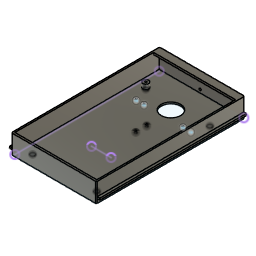
new_Backplate v28 (Autodesk Fusion 360 design; units mm, degrees)
Autodesk Fusion 360 part; units mm, degrees
sketch "Sketch1" plane through (0, 0, 0) normal (0, 0, 1) x (1, 0, 0)
  line L0 (0, 0) -> (109, 0)
  line L1 (109, 0) -> (109, 190)
  line L2 (109, 190) -> (0, 190)
  line L3 (0, 190) -> (0, 0)
  dimension "d1" = 190
  dimension "d2" = 109
  constraint horizontal L0
  constraint vertical L1
  constraint horizontal L2
  constraint vertical L3
  constraint coincident L0.start L3.end
  measures "d1" distance of L0.start L2.end
  measures "d2" distance of L0.start L0.end
extrude "Extrude1" add sketch "Sketch1" along normal blind 18.5 makes body 1
sketch "Sketch2" plane through (0, 0, 18.5) normal (0, 0, 1) x (-1, 0, 0)
  line L0 (0, -190) -> (0, 0)
  line L1 (0, 0) -> (-109, 0)
  line L2 (-109, 0) -> (-109, -190)
  line L3 (-109, -190) -> (0, -190)
  line L4 (-2, -187.5) -> (-107, -187.5)
  line L5 (-107, -187.5) -> (-107, -2.5)
  line L6 (-107, -2.5) -> (-2, -2.5)
  line L7 (-2, -2.5) -> (-2, -187.5)
  dimension "d5" = 2.5
  dimension "d6" = 2.5
  dimension "d7" = 2
  dimension "d8" = 2
  constraint horizontal L4
  constraint vertical L5
  constraint horizontal L6
  constraint vertical L7
  measures "d5" distance of L3 L4
  measures "d6" distance of L1 L6
  measures "d7" distance of L0 L7
  measures "d8" distance of L2 L5
extrude "Extrude2" cut sketch "Sketch2" against normal blind 16.5 contours L4 L5 L6 L7 bodies 1
chamfer "Chamfer1" distance 1 angle 45 4 edges at (0, 190, 9.25) (109, 190, 9.25) (0, 0, 9.25) (109, 0, 9.25) on bodies 1
sketch "Sketch3" plane through (0, 0, 2) normal (0, 0, 1) x (-1, 0, 0)
  line L0 (-2, -2.5) -> (-107, -2.5)
  line L1 (-107, -2.5) -> (-107, -187.5)
  line L2 (-107, -187.5) -> (-2, -187.5)
  line L3 (-2, -187.5) -> (-2, -2.5)
  circle A0 centre (-13.3, -159) radius 1.25
  circle A1 centre (-95.5, -159) radius 1.25
  circle A2 centre (-13.3, -14) radius 1.25
  circle A3 centre (-95.5, -14) radius 1.25
  dimension "d12" = 2.5
  dimension "d13" = 2.5
  dimension "d14" = 2.5
  dimension "d15" = 2.5
  dimension "d17" = 11.3
  dimension "d18" = 11.5
  dimension "d20" = 11.5
  dimension "d21" = 11.5
  dimension "d22" = 11.3
  dimension "d23" = 11.5
  dimension "d26" = 145
  dimension "d27" = 145
  measures "d12" diameter of A3
  measures "d13" diameter of A2
  measures "d14" diameter of A1
  measures "d15" diameter of A0
  measures "d17" distance of L3 A0.centre
  measures "d18" distance of L1 A1.centre
  measures "d20" distance of L1 A3.centre
  measures "d21" distance of L0 A3.centre
  measures "d22" distance of L3 A2.centre
  measures "d23" distance of L0 A2.centre
  measures "d26" distance of A0.centre A2.centre
  measures "d27" distance of A1.centre A3.centre
extrude "Extrude3" cut sketch "Sketch3" against normal blind 2.5 contours A0 | A1 | A2 | A3 bodies 1
sketch "Sketch4" plane through (0, 0, 0) normal (0, 0, -1) x (1, 0, 0)
  circle A0 centre (95.5, -14) radius 1.25
  circle A1 centre (95.5, -159) radius 1.25
  circle A2 centre (13.3, -14) radius 1.25
  circle A3 centre (13.3, -159) radius 1.25
  line L0 (109, -1) -> (108, 0)
  line L1 (108, 0) -> (1, 0)
  line L2 (1, 0) -> (0, -1)
  line L3 (0, -1) -> (0, -189)
  line L4 (0, -189) -> (1, -190)
  line L5 (1, -190) -> (108, -190)
  line L6 (108, -190) -> (109, -189)
  line L7 (109, -189) -> (109, -1)
  line L8 (6, -177.5) -> (6, -75)
  line L9 (103, -75) -> (103, -177.5)
  line L10 (8.5, -175) -> (8.5, -75)
  line L11 (100.5, -75) -> (100.5, -175)
  line L12 (103, -75) -> (100.5, -75)
  line L13 (8.5, -75) -> (6, -75)
  line L14 (100.5, -175) -> (100.5, -177.5)
  line L15 (8.5, -175) -> (8.5, -177.5)
  line L16 (103, -177.5) -> (103, -190)
  line L17 (6, -190) -> (6, -177.5)
  line L18 (100.5, -177.5) -> (100.5, -190)
  line L19 (103, -190) -> (100.5, -190)
  line L20 (8.5, -177.5) -> (8.5, -190)
  line L21 (6, -190) -> (8.5, -190)
  line L22 (8.5, -190) -> (6, -190)
  dimension "d28" = 6
  dimension "d29" = 6
  dimension "d32" = 2.5
  dimension "d34" = 2.5
  dimension "d38" = 115
  dimension "d39" = 115
  constraint vertical L8
  constraint vertical L9
  constraint vertical L10
  constraint vertical L11
  constraint perpendicular L11 L12
  constraint perpendicular L8 L13
  constraint coincident L5 L16.end
  constraint perpendicular L5 L16
  constraint coincident L5 L17.start
  constraint perpendicular L5 L17
  constraint coincident L5 L18.end
  constraint perpendicular L5 L18
  constraint coincident L5 L20.end
  constraint perpendicular L5 L20
  measures "d28" distance of L3 L8
  measures "d29" distance of L7 L9
  measures "d32" distance of L8 L10
  measures "d34" distance of L9 L11
  measures "d38" distance of L5 L11.start
  measures "d39" distance of L5 L10.end
sketch "Sketch5" plane through (0, 0, 2) normal (0, 0, 1) x (-1, 0, 0)
  circle A0 centre (-95.5, -14) radius 1.25
  circle A1 centre (-95.5, -159) radius 1.25
  circle A2 centre (-13.3, -14) radius 1.25
  circle A3 centre (-13.3, -159) radius 1.25
  line L0 (-2, -2.5) -> (-107, -2.5)
  line L1 (-107, -2.5) -> (-107, -187.5)
  line L2 (-107, -187.5) -> (-2, -187.5)
  line L3 (-2, -187.5) -> (-2, -2.5)
  circle A4 centre (-54.5, -150) radius 12.5
  line L4 (-109, -189) -> (-109, -1)
  line L5 (-1, -190) -> (-108, -190)
  dimension "d42" = 54.5
  dimension "d43" = 40
  dimension "d44" = 25
  measures "d42" distance of A4.centre L4
  measures "d43" distance of A4.centre L5
  measures "d44" diameter of A4
extrude "Extrude6" cut sketch "Sketch5" against normal blind 2.5 contours A4 bodies 1
ref_plane "WorkPlane1" through (42, 0, 0) normal (1, 0, 0) x (0, 1, 0)
sketch "Sketch16" plane through (42, 0, 0) normal (1, 0, 0) x (0, 1, 0)
  line L0 (57.55, 0.0575) -> (53.25, 0.0575)
  line L1 (50, -5.5717) -> (60.8, -5.5717)
  line L2 (60.8, -5.5717) -> (57.55, 0.0575)
  line L3 (53.25, 0.0575) -> (50, -5.5717)
  dimension "d74" = 120
  dimension "d75" = 120
  dimension "d76" = 10.8
  dimension "d77" = 6.5
  dimension "d90" = 50
  constraint horizontal L0
  constraint horizontal L1
  measures "d74" angle of L0 L2
  measures "d75" angle of L0 L3
  measures "d76" distance of L1.start L1.end
  measures "d77" distance of L1.end L0.start
  measures "d90" horizontal distance of L1.start origin
extrude "Extrude16" add sketch "Sketch16" along normal blind 25 separate body makes body 2
sketch "Sketch17" plane through (0, 0, 0) normal (0, 0, -1) x (1, 0, 0)
  circle A0 centre (13.3, -14) radius 1.25
  circle A1 centre (95.5, -14) radius 1.25
  line L0 (1, -190) -> (108, -190)
  line L1 (108, -190) -> (109, -189)
  line L2 (109, -189) -> (109, -1)
  line L3 (109, -1) -> (108, 0)
  line L4 (108, 0) -> (1, 0)
  line L5 (1, 0) -> (0, -1)
  line L6 (0, -1) -> (0, -189)
  line L7 (0, -189) -> (1, -190)
  circle A2 centre (13.3, -159) radius 1.25
  circle A3 centre (95.5, -159) radius 1.25
  circle A4 centre (54.5, -150) radius 12.5
  line L8 (100.5, -182.7) -> (8.5, -182.7)
  line L9 (8.5, -182.7) -> (8.5, -180.7)
  line L10 (8.5, -180.7) -> (100.5, -180.7)
  line L11 (100.5, -180.7) -> (100.5, -182.7)
  dimension "d81" = 2
  constraint horizontal L8
  constraint vertical L9
  constraint horizontal L10
  constraint vertical L11
  measures "d81" distance of L8 L10
sketch "Sketch20" plane through (0, 0, 2) normal (0, 0, 1) x (-1, 0, 0)
  circle A0 centre (-54.5, -150) radius 12.5
  circle A1 centre (-95.5, -14) radius 1.25
  circle A2 centre (-95.5, -159) radius 1.25
  circle A3 centre (-13.3, -14) radius 1.25
  circle A4 centre (-13.3, -159) radius 1.25
  line L0 (-2, -2.5) -> (-107, -2.5)
  line L1 (-107, -2.5) -> (-107, -187.5)
  line L2 (-107, -187.5) -> (-2, -187.5)
  line L3 (-2, -187.5) -> (-2, -2.5)
  circle A5 centre (-13.3, -159) radius 3.75
  circle A6 centre (-95.5, -159) radius 3.75
  circle A7 centre (-13.3, -14) radius 3.75
  circle A8 centre (-95.5, -14) radius 3.75
  dimension "d91" = 7.5
  dimension "d92" = 7.5
  dimension "d93" = 7.5
  dimension "d94" = 7.5
  constraint concentric A4 A5
  constraint concentric A2 A6
  constraint concentric A3 A7
  constraint concentric A1 A8
  measures "d91" diameter of A8
  measures "d92" diameter of A7
  measures "d93" diameter of A5
  measures "d94" diameter of A6
extrude "Extrude20" add sketch "Sketch20" along normal blind 6 contours A5 | A6 | A7 | A8 bodies 1
sketch "Sketch21" plane through (0, 0, 18.5) normal (0, 0, 1) x (-1, 0, 0)
  line L0 (-107, -187.5) -> (-107, -2.5)
  line L1 (-107, -2.5) -> (-2, -2.5)
  line L2 (-2, -2.5) -> (-2, -187.5)
  line L3 (-2, -187.5) -> (-107, -187.5)
  line L4 (-108, 0) -> (-109, -1)
  line L5 (-109, -1) -> (-109, -189)
  line L6 (-109, -189) -> (-108, -190)
  line L7 (-108, -190) -> (-1, -190)
  line L8 (-1, -190) -> (0, -189)
  line L9 (0, -189) -> (0, -1)
  line L10 (0, -1) -> (-1, 0)
  line L11 (-1, 0) -> (-108, 0)
  line L12 (-1, -190) -> (-108, -190)
  line L13 (-109, -179) -> (-109, -1)
  line L14 (-108, 0) -> (-1, 0)
  line L15 (0, -1) -> (0, -179)
  line L16 (-108, 0) -> (-109, -1)
  line L17 (0, -1) -> (-1, 0)
  line L18 (0, -189) -> (-1, -190)
  line L19 (-108, -190) -> (-109, -189)
  line L20 (-2, -187.5) -> (-107, -187.5)
  line L21 (-107, -187.5) -> (-107, -2.5)
  line L22 (-107, -2.5) -> (-2, -2.5)
  line L23 (-2, -2.5) -> (-2, -187.5)
  constraint horizontal L12
  constraint vertical L13
  constraint horizontal L14
  constraint vertical L15
  constraint coincident L4.start L11.end
  constraint coincident L4.end L5.start
  constraint coincident L9.end L10.start
  constraint coincident L10.end L11.start
  constraint coincident L8.end L9.start
  constraint coincident L7.end L8.start
  constraint coincident L6.end L7.start
  constraint coincident L5.end L6.start
  constraint horizontal L20
  constraint vertical L21
  constraint horizontal L22
  constraint vertical L23
  constraint coincident L0.end L1.start
  constraint coincident L2.end L3.start
extrude "Extrude21" add sketch "Sketch21" along normal blind 6 bodies 1
sketch "Sketch23" plane through (0, 187.5, 0) normal (0, -1, 0) x (1, 0, 0)
  line L0 (2, 24.5) -> (2, 2)
  line L1 (2, 2) -> (107, 2)
  line L2 (107, 2) -> (107, 24.5)
  line L3 (107, 24.5) -> (2, 24.5)
  line L4 (2, 24.5) -> (107, 24.5)
  line L5 (107, 24.5) -> (107, 22)
  line L6 (107, 22) -> (2, 22)
  line L7 (2, 22) -> (2, 24.5)
  constraint horizontal L4
  constraint vertical L5
  constraint horizontal L6
  constraint vertical L7
  constraint coincident L2 L5.end
  constraint coincident L0.start L3.end
extrude "Extrude22" add sketch "Sketch23" along normal blind 7.25 contours L0 L2 L3 L4 L5 L6 L7 bodies 1
sketch "Sketch24" plane through (0, 0, 0) normal (0, 0, -1) x (1, 0, 0)
  circle A0 centre (95.5, -14) radius 1.25
  circle A1 centre (13.3, -14) radius 1.25
  circle A2 centre (13.3, -159) radius 1.25
  circle A3 centre (95.5, -159) radius 1.25
  circle A4 centre (54.5, -150) radius 12.5
  line L0 (1, -190) -> (108, -190)
  line L1 (108, -190) -> (109, -189)
  line L2 (109, -189) -> (109, -1)
  line L3 (109, -1) -> (108, 0)
  line L4 (108, 0) -> (1, 0)
  line L5 (1, 0) -> (0, -1)
  line L6 (0, -1) -> (0, -189)
  line L7 (0, -189) -> (1, -190)
  circle A5 centre (13.3, -14) radius 2.75
  circle A6 centre (95.5, -14) radius 2.75
  circle A7 centre (95.5, -159) radius 2.75
  circle A8 centre (13.3, -159) radius 2.75
  circle A9 centre (90, -140) radius 1.2
  circle A10 centre (80, -140) radius 1.2
  circle A11 centre (30, -140) radius 1.2
  circle A12 centre (20, -140) radius 1.2
  circle A13 centre (55, -118.5) radius 1.2
  circle A14 centre (55, -104.5) radius 1.2
  line L8 (2, -2.5) -> (2, -187.5)
  line L9 (42, -60.8) -> (67, -60.8)
  dimension "d102" = 2.4
  dimension "d103" = 2.4
  dimension "d104" = 2.4
  dimension "d105" = 2.4
  dimension "d106" = 5.5
  dimension "d107" = 5.5
  dimension "d108" = 5.5
  dimension "d109" = 5.5
  dimension "d114" = 2.4
  dimension "d115" = 2.4
  dimension "d117" = 14
  dimension "d128" = 53
  dimension "d129" = 53
  dimension "d130" = 43.7
  constraint concentric A1 A5
  constraint concentric A0 A6
  constraint concentric A3 A7
  constraint concentric A2 A8
  measures "d102" diameter of A9
  measures "d103" diameter of A10
  measures "d104" diameter of A11
  measures "d105" diameter of A12
  measures "d106" diameter of A8
  measures "d107" diameter of A7
  measures "d108" diameter of A6
  measures "d109" diameter of A5
  measures "d114" diameter of A14
  measures "d115" diameter of A13
  measures "d117" vertical distance of A13.centre A14.centre
  measures "d128" distance of A14.centre L8
  measures "d129" distance of A13.centre L8
  measures "d130" distance of A14.centre L9
extrude "Extrude23" cut sketch "Sketch24" against normal blind 6 contours A5 | A6 | A7 | A8 bodies 1
extrude "Extrude24" cut sketch "Sketch24" against normal blind 2 contours A9 | A10 | A11 | A12 | A13 | A14 bodies 1
sketch "Sketch25" plane through (0, 0, 0) normal (-1, 0, 0) x (0, -1, 0)
  line L0 (-1, 24.5) -> (-189, 24.5)
  line L1 (-189, 0) -> (-1, 0)
  line L2 (-1, 7.45) -> (-184, 7.45)
  line L3 (-184, 7.45) -> (-184, 5.2)
  line L4 (-184, 5.2) -> (-1, 5.2)
  line L5 (-1, 5.2) -> (-1, 7.45)
  line L6 (-16.75, 0) -> (-11.25, 0)
  dimension "d121" = 2.25
  dimension "d132" = 5.2
  constraint horizontal L2
  constraint vertical L3
  constraint horizontal L4
  constraint vertical L5
  measures "d121" distance of L2 L4
  measures "d132" distance of L4 L6
extrude "Extrude25" add sketch "Sketch25" along normal blind 3.3 bodies 1
sketch "Sketch26" plane through (109, 0, 0) normal (1, 0, 0) x (0, 1, 0)
  line L0 (1, 24.5) -> (1, 0)
  line L1 (1, 0) -> (189, 0)
  line L2 (189, 0) -> (189, 24.5)
  line L3 (189, 24.5) -> (1, 24.5)
  line L4 (1, 7.45) -> (189, 7.45)
  line L5 (189, 7.45) -> (189, 5.2)
  line L6 (189, 5.2) -> (1, 5.2)
  line L7 (1, 5.2) -> (1, 7.45)
  line L8 (189, 0) -> (1, 0)
  dimension "d124" = 2.25
  dimension "d131" = 5.2
  constraint horizontal L4
  constraint vertical L5
  constraint horizontal L6
  constraint vertical L7
  constraint coincident L2 L5.end
  constraint coincident L0 L4.start
  measures "d124" distance of L4 L6
  measures "d131" distance of L6 L8
extrude "Extrude26" add sketch "Sketch26" along normal blind 3.3 contours L0 L2 L4 L5 L6 L7 bodies 1
sketch "Sketch27" plane through (0, 190, 0) normal (0, 1, 0) x (-1, 0, 0)
  line L0 (-108, 24.5) -> (-108, 0)
  line L1 (-108, 0) -> (-1, 0)
  line L2 (-1, 0) -> (-1, 24.5)
  line L3 (-1, 24.5) -> (-108, 24.5)
  circle A0 centre (-54.5, 6) radius 1.375
  point P0 (-54.5, 0)
  dimension "d133" = 2.75
  dimension "d134" = 6
  dimension "d135" = 53.5
  measures "d133" diameter of A0
  measures "d134" vertical distance of A0.centre P0
  measures "d135" distance of L0 A0.centre
extrude "Extrude27" cut sketch "Sketch27" against normal blind 3 contours A0 bodies 1
